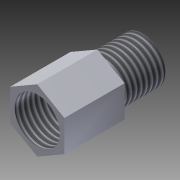
# Autodesk Inventor part: Standoff
Saved by Autodesk Inventor 2015 (Build 190159000, 159)
## iProperties
Created: 2017-01-16
Part Number: Standoff
Material: Generic
Document SubType Name: Modeling
Designer: Per
Density: 1 g/cm^3
Appearance: PTFE
Author: Per
Autodesk Inventor part; units mm, degrees
ref_plane "YZ Plane" through (0, 0, 0) normal (1, 0, 0) x (0, 1, 0)
ref_plane "XZ Plane" through (0, 0, 0) normal (0, 1, 0) x (-1, 0, 0)
ref_plane "XY Plane" through (0, 0, 0) normal (0, 0, 1) x (1, 0, 0)
sketch "Sketch1" plane through (0, 0, 0) normal (0, 1, 0) x (-1, 0, 0)
  line L0 (1.7985, -1.0383) -> (0, -2.0767)
  line L1 (0, -2.0767) -> (-1.7985, -1.0383)
  line L2 (-1.7985, -1.0383) -> (-1.7985, 1.0383)
  line L3 (-1.7985, 1.0383) -> (0, 2.0767)
  line L4 (0, 2.0767) -> (1.7985, 1.0383)
  line L5 (1.7985, 1.0383) -> (1.7985, -1.0383)
  point P0 (0, 0)
  point P1 (0, 0)
  point P2 (0, 0)
  constraints: 12 end point, 1 coincident, 13 other
extrude "Extrusion1" add sketch "Sketch1" along normal blind 4
sketch "Sketch2" plane through (0, 4, 0) normal (0, 1, 0) x (1, 0, 0)
  circle A0 centre (0, 0) radius 1.5
  dimension "d3" = 3
  constraints: 1 centre point, 1 coincident
  measures "d3" diameter of A0
extrude "Extrusion2" add sketch "Sketch2" along normal blind 3
thread "Thread1" size "M3x0.35" class "6g" standard "ANSI Metric M Profile" full length
sketch "Sketch3" plane through (0, 0, 0) normal (0, -1, 0) x (1, 0, 0)
  circle A0 centre (0, 0) radius 1.5
  dimension "d8" = 3
  constraints: 1 centre point, 1 coincident
  measures "d8" diameter of A0
extrude "Extrusion3" cut sketch "Sketch3" against normal blind 3
thread "Thread2" size "M3x0.35" class "6H" standard "ANSI Metric M Profile" full length
body "Solid1"
